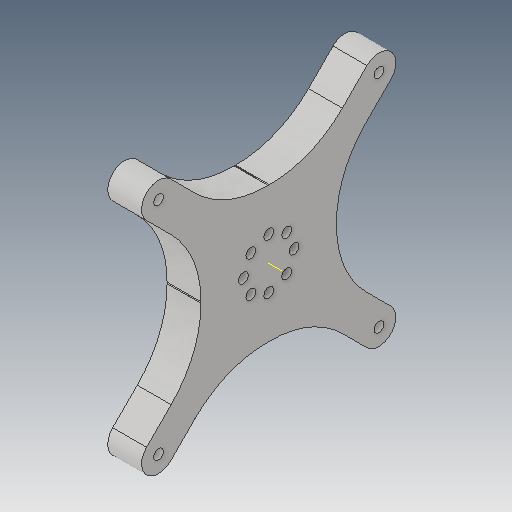
# Autodesk Inventor part: ThrusterMountv2(3)
Saved by Autodesk Inventor 2018 (Build 220112000, 112)
## iProperties
Created: 2019-02-16
Part Number: ThrusterMountv2(3)
Material: Generic
Document SubType Name: Modeling
Designer: anirudh
Density: 1 g/cm^3
Appearance: Default
Mass: 71.9019 g
Surface Area: 161.668 cm^2
Volume: 71.9019 cm^3
Author: anirudh
Autodesk Inventor part; units mm, degrees
ref_plane "YZ Plane" through (0, 0, 0) normal (1, 0, 0) x (0, 1, 0)
ref_plane "XZ Plane" through (0, 0, 0) normal (0, 1, 0) x (-1, 0, 0)
ref_plane "XY Plane" through (0, 0, 0) normal (0, 0, 1) x (1, 0, 0)
sketch "Sketch1" plane through (0, 0, 0) normal (1, 0, 0) x (0, 1, 0)
  circle A0 centre (82.55, 0) radius 1.85
  circle A1 centre (82.55, -82.55) radius 1.85
  circle A2 centre (0, 0) radius 1.85
  circle A3 centre (0, -82.55) radius 1.85
  line L0 (82.55, 0) -> (91.4656, 0) construction
  line L1 (82.55, -82.55) -> (88.8543, -82.55) construction
  arc A4 (54.1751, -19.3947) -> (28.3749, -19.3947) centre (41.275, -41.275) ccw
  arc A5 (19.3947, -28.3749) -> (19.3947, -54.1751) centre (41.275, -41.275) ccw
  arc A6 (28.3749, -63.1553) -> (54.1751, -63.1553) centre (41.275, -41.275) ccw
  arc A7 (63.1553, -54.1751) -> (63.1553, -28.3749) centre (41.275, -41.275) ccw
  arc A8 (87.0401, -4.4901) -> (78.0599, 4.4901) centre (82.55, 0) ccw
  arc A9 (4.4901, 4.4901) -> (-4.4901, -4.4901) centre (0, 0) ccw
  arc A10 (-4.4901, -78.0599) -> (4.4901, -87.0401) centre (0, -82.55) ccw
  arc A11 (78.0599, -87.0401) -> (87.0401, -78.0599) centre (82.55, -82.55) ccw
  line L2 (78.0599, 4.4901) -> (54.1751, -19.3947)
  line L3 (87.0401, -4.4901) -> (63.1553, -28.3749)
  line L4 (87.0401, -78.0599) -> (63.1553, -54.1751)
  line L5 (78.0599, -87.0401) -> (54.1751, -63.1553)
  line L6 (19.3947, -54.1751) -> (-4.4901, -78.0599)
  line L7 (28.3749, -63.1553) -> (4.4901, -87.0401)
  line L8 (19.3947, -28.3749) -> (-4.4901, -4.4901)
  line L9 (4.4901, 4.4901) -> (28.3749, -19.3947)
  circle A12 centre (41.275, -31.775) radius 1.85
  circle A13 centre (50.775, -41.275) radius 1.85
  circle A14 centre (41.275, -50.775) radius 1.85
  circle A15 centre (31.775, -41.275) radius 1.85
  constraints: 20 end point, 16 centre point, 16 point on circle, 6 coincident, 2 horizontal, 1 parallel, 1 perpendicular, 1 tangent
extrude "Extrusion1" add sketch "Sketch1" along normal blind 7.9375
sketch "Sketch2" plane through (0, 0, 0) normal (-1, 0, 0) x (0, 0, 1)
  circle A0 centre (-82.55, 82.55) radius 1.85 projected
  circle A1 centre (-82.55, 82.55) radius 6.35
  arc A2 (4.4901, 78.0599) -> (-4.4901, 87.0401) centre (0, 82.55) ccw projected
  circle A3 centre (0, 82.55) radius 6.35
  circle A4 centre (-82.55, 82.55) radius 1.85
  circle A5 centre (0, 82.55) radius 1.85
  circle A6 centre (0, 0) radius 1.85
  circle A7 centre (0, 0) radius 6.35
  circle A8 centre (-82.55, 0) radius 1.85 projected
  circle A9 centre (-82.55, 0) radius 1.85
  circle A10 centre (-82.55, 0) radius 6.35
  dimension "d24" = 3.7
  constraints: 8 centre point, 8 coincident
  measures "d24" diameter of A4
extrude "Extrusion2" add sketch "Sketch2" along normal blind 7.9375
sketch "Sketch3" plane through (7.9375, 0, 0) normal (1, 0, 0) x (0, 0, -1)
  arc A0 (-4.4901, 4.4901) -> (4.4901, -4.4901) centre (0, 0) ccw
  arc A1 (4.4901, 87.0401) -> (-4.4901, 78.0599) centre (0, 82.55) ccw projected
  arc A2 (4.4901, 87.0401) -> (-4.4901, 78.0599) centre (0, 82.55) ccw
  arc A3 (87.0401, 78.0599) -> (78.0599, 87.0401) centre (82.55, 82.55) ccw projected
  arc A4 (87.0401, 78.0599) -> (78.0599, 87.0401) centre (82.55, 82.55) ccw
  arc A5 (78.0599, -4.4901) -> (87.0401, 4.4901) centre (82.55, 0) ccw projected
  arc A6 (78.0599, -4.4901) -> (87.0401, 4.4901) centre (82.55, 0) ccw
  line L0 (4.4901, 78.0599) -> (0, 73.5697)
  line L1 (-4.4901, 78.0599) -> (19.3947, 54.1751) projected
  line L2 (-4.4901, 78.0599) -> (0, 73.5697)
  line L3 (0, 73.5697) -> (8.9803, 82.55)
  line L4 (28.3749, 63.1553) -> (4.4901, 87.0401) projected
  line L5 (8.9803, 82.55) -> (4.4901, 87.0401)
  line L6 (78.0599, 78.0599) -> (73.5697, 82.55)
  line L7 (73.5697, 82.55) -> (78.0599, 87.0401)
  line L8 (78.0599, 87.0401) -> (73.5697, 82.55)
  line L9 (73.5697, 82.55) -> (82.55, 73.5697)
  line L10 (63.1553, 54.1751) -> (87.0401, 78.0599) projected
  line L11 (82.55, 73.5697) -> (87.0401, 78.0599)
  line L12 (4.4901, 4.4901) -> (0, 8.9803)
  line L13 (19.3947, 28.3749) -> (-4.4901, 4.4901) projected
  line L14 (0, 8.9803) -> (-4.4901, 4.4901)
  line L15 (-4.4901, 4.4901) -> (0, 8.9803)
  line L16 (0, 8.9803) -> (8.9803, 0)
  line L17 (4.4901, -4.4901) -> (28.3749, 19.3947) projected
  line L18 (8.9803, 0) -> (4.4901, -4.4901)
  line L19 (78.0599, 4.4901) -> (73.5697, 0)
  line L20 (73.5697, 0) -> (78.0599, -4.4901)
  line L21 (78.0599, 4.4901) -> (82.55, 8.9803)
  line L22 (87.0401, 4.4901) -> (63.1553, 28.3749) projected
  line L23 (82.55, 8.9803) -> (87.0401, 4.4901)
  constraints: 37 end point, 14 tangent, 13 point on line, 10 point on circle, 9 perpendicular, 4 centre point, 4 coincident, 2 collinear, 2 midpoint, 1 parallel
extrude "Extrusion3" cut sketch "Sketch3" against normal blind 3.175
fillet "Fillet4" radius 38.1 8 edges at (3.9688, 63.1553, -28.3749) (3.9688, 63.1553, -54.1751) (3.9688, 54.1751, -19.3947) (3.9688, 28.3749, -19.3947) (3.9688, 54.1751, -63.1553) (3.9688, 28.3749, -63.1553) (3.9688, 19.3947, -28.3749) (3.9688, 19.3947, -54.1751)
ref_plane "Work Plane1" through (3.9688, 0, 0) normal (1, 0, 0) x (0, 0, -1)
sketch "Sketch6" plane through (3.9688, 0, 0) normal (1, 0, 0) x (0, 0, -1)
  line L0 (18.1155, 56.3523) -> (26.1977, 64.4345) projected
  line L1 (26.1977, 64.4345) -> (18.1155, 56.3523)
  line L2 (36.525, 46.025) -> (18.1155, 56.3523) projected
  line L3 (18.1155, 56.3523) -> (36.525, 46.025)
  line L4 (36.525, 46.025) -> (26.1977, 64.4345)
  line L5 (56.3523, 64.4345) -> (46.025, 46.025) projected
  line L6 (56.3523, 64.4345) -> (46.025, 46.025)
  line L7 (46.025, 46.025) -> (64.4345, 56.3523) projected
  line L8 (46.025, 46.025) -> (64.4345, 56.3523)
  line L9 (56.3523, 64.4345) -> (64.4345, 56.3523) projected
  line L10 (64.4345, 56.3523) -> (56.3523, 64.4345)
  line L11 (18.1155, 26.1977) -> (26.1977, 18.1155) projected
  line L12 (18.1155, 26.1977) -> (26.1977, 18.1155)
  line L13 (36.525, 36.525) -> (26.1977, 18.1155) projected
  line L14 (26.1977, 18.1155) -> (36.525, 36.525)
  line L15 (36.525, 36.525) -> (18.1155, 26.1977)
  line L16 (56.3523, 18.1155) -> (46.025, 36.525) projected
  line L17 (64.4345, 26.1977) -> (56.3523, 18.1155) projected
  line L18 (56.3523, 18.1155) -> (64.4345, 26.1977)
  line L19 (46.025, 36.525) -> (64.4345, 26.1977) projected
  line L20 (64.4345, 26.1977) -> (46.025, 36.525)
  line L21 (46.025, 36.525) -> (56.3523, 18.1155)
  point P0 (0, 0)
  constraints: 24 end point, 9 collinear
extrude "Extrusion5" add sketch "Sketch6" along normal blind 1.27 and the other way blind 3.9688
sketch "Sketch10" plane through (7.9375, 0, 0) normal (1, 0, 0) x (0, 0, -1)
  circle A0 centre (50.775, 41.275) radius 1.85 projected
  circle A1 centre (50.775, 41.275) radius 1.85
  circle A2 centre (41.275, 31.775) radius 1.85 projected
  circle A3 centre (41.275, 31.775) radius 1.85
  circle A4 centre (31.775, 41.275) radius 1.85 projected
  circle A5 centre (31.775, 41.275) radius 1.85
  circle A6 centre (41.275, 50.775) radius 1.85 projected
  circle A7 centre (41.275, 50.775) radius 1.85
  line L0 (82.55, 8.9803) -> (77.8311, 13.6992) projected
  line L1 (68.8508, 4.7189) -> (73.5697, 0) projected
  line L2 (82.55, 8.9803) -> (73.5697, 0)
  line L3 (8.9803, 0) -> (13.6992, 4.7189) projected
  line L4 (4.7189, 13.6992) -> (0, 8.9803) projected
  line L5 (8.9803, 0) -> (0, 8.9803)
  line L6 (82.55, 73.5697) -> (73.5697, 82.55) projected
  line L7 (82.55, 73.5697) -> (73.5697, 82.55)
  line L8 (13.6992, 77.8311) -> (8.9803, 82.55) projected
  line L9 (8.9803, 82.55) -> (0, 73.5697)
  line L10 (77.8311, 68.8508) -> (82.55, 73.5697) projected
  line L11 (82.55, 73.5697) -> (77.8311, 68.8508)
  line L12 (73.5697, 82.55) -> (68.8508, 77.8311) projected
  line L13 (73.5697, 82.55) -> (68.8508, 77.8311)
  line L14 (8.9803, 82.55) -> (0, 73.5697) projected
  line L15 (8.9803, 82.55) -> (13.6992, 77.8311)
  line L16 (0, 73.5697) -> (4.7189, 68.8508) projected
  line L17 (0, 73.5697) -> (4.7189, 68.8508)
  line L18 (0, 8.9803) -> (8.9803, 0) projected
  line L19 (8.9803, 0) -> (13.6992, 4.7189)
  line L20 (0, 8.9803) -> (4.7189, 13.6992)
  line L21 (73.5697, 0) -> (82.55, 8.9803) projected
  line L22 (73.5697, 0) -> (68.8508, 4.7189)
  line L23 (82.55, 8.9803) -> (77.8311, 13.6992)
  arc A8 (41.021, 15.8763) -> (41.529, 15.8763) centre (41.275, 41.275) ccw projected
  line L24 (41.529, 15.8763) -> (41.021, 15.8763)
  arc A9 (15.8763, 41.529) -> (15.8763, 41.021) centre (41.275, 41.275) ccw projected
  line L25 (15.8763, 41.021) -> (15.8763, 41.529)
  arc A10 (41.529, 66.6737) -> (41.021, 66.6737) centre (41.275, 41.275) ccw projected
  line L26 (41.529, 66.6737) -> (41.021, 66.6737)
  arc A11 (66.6737, 41.021) -> (66.6737, 41.529) centre (41.275, 41.275) ccw projected
  line L27 (66.6737, 41.021) -> (66.6737, 41.529)
  arc A12 (68.8508, 4.7189) -> (41.529, 15.8763) centre (41.91, -22.2218) ccw projected
  arc A13 (68.8508, 4.7189) -> (41.529, 15.8763) centre (41.91, -22.2218) ccw
  arc A14 (41.021, 15.8763) -> (13.6992, 4.7189) centre (40.64, -22.2218) ccw
  arc A15 (4.7189, 13.6992) -> (15.8763, 41.021) centre (-23.1549, 41.021) ccw
  arc A16 (15.8763, 41.529) -> (4.7189, 68.8508) centre (-22.2218, 41.91) ccw projected
  arc A17 (15.8763, 41.529) -> (4.7189, 68.8508) centre (-22.2218, 41.91) ccw
  arc A18 (13.6992, 77.8311) -> (41.021, 66.6737) centre (40.64, 104.7718) ccw
  arc A19 (41.529, 66.6737) -> (68.8508, 77.8311) centre (41.91, 104.7718) ccw projected
  arc A20 (41.529, 66.6737) -> (68.8508, 77.8311) centre (41.91, 104.7718) ccw
  arc A21 (77.8311, 68.8508) -> (66.6737, 41.529) centre (104.7718, 41.91) ccw projected
  arc A22 (77.8311, 68.8508) -> (66.6737, 41.529) centre (104.7718, 41.91) ccw
  arc A23 (66.6737, 41.021) -> (77.8311, 13.6992) centre (104.7718, 40.64) ccw
  point P0 (0, 0)
  constraints: 32 end point, 16 point on circle, 12 centre point, 8 collinear, 4 coincident, 3 perpendicular, 3 tangent, 2 horizontal, 2 vertical, 1 point on line
extrude "Extrusion8" cut sketch "Sketch10" against normal blind 3.175
sketch "Sketch11" plane through (7.9375, 41.021, -66.6737) normal (0, 0, 1) x (1, 0, 0)
  line L0 (0, 0.508) -> (-3.175, 0.508) projected
  line L1 (-3.175, 0) -> (0, 0) projected
  line L2 (0, 0.508) -> (-3.175, 0.508)
  line L3 (-3.175, 0.508) -> (-3.175, 0)
  line L4 (-3.175, 0) -> (0, 0)
  line L5 (0, 0) -> (0, 0.508)
  point P0 (-7.9375, -41.021)
  constraints: 8 end point, 2 parallel, 1 horizontal, 1 perpendicular
extrude "Extrusion9" cut sketch "Sketch11" along normal blind 50.8 and the other way blind 25.4
sketch "Sketch12" plane through (7.9375, 15.8763, -41.021) normal (0, 1, 0) x (1, 0, 0)
  line L0 (0, 0) -> (0, 0.508) projected
  line L1 (-3.175, 0.508) -> (0, 0.508) projected
  line L2 (0, 0) -> (-3.175, 0)
  line L3 (-3.175, 0) -> (-3.175, 0.508)
  line L4 (-3.175, 0.508) -> (0, 0.508)
  line L5 (0, 0.508) -> (0, 0)
  point P0 (-7.9375, -41.021)
  constraints: 8 end point, 2 parallel, 1 horizontal, 1 perpendicular
extrude "Extrusion10" cut sketch "Sketch12" along normal blind 53.975 and the other way blind 7.9375
sketch "Sketch13" plane through (4.7625, 0, 0) normal (1, 0, 0) x (0, 0, -1)
  line L0 (41.275, 41.275) -> (41.275, 43.8729)
  circle A0 centre (34.5575, 34.5575) radius 1.85
  circle A1 centre (34.5575, 47.9925) radius 1.85
  circle A2 centre (47.9925, 34.5575) radius 1.85
  circle A3 centre (47.9925, 47.9925) radius 1.85
  point P0 (0, 0)
  point P1 (41.275, 50.775)
  point P2 (41.275, 31.775)
  point P3 (50.775, 41.275)
  constraints: 4 centre point, 2 end point, 1 vertical
extrude "Extrusion12" cut sketch "Sketch13" against normal blind 24.5364
sketch "Sketch15" plane through (0, 0, 0) normal (-1, 0, 0) x (0, 0, 1)
  circle A0 centre (-34.5575, 34.5575) radius 1.85 projected
  circle A1 centre (-34.5575, 34.5575) radius 1.85
  circle A2 centre (-34.5575, 47.9925) radius 1.85 projected
  circle A3 centre (-34.5575, 47.9925) radius 1.85
  circle A4 centre (-47.9925, 47.9925) radius 1.85 projected
  circle A5 centre (-47.9925, 47.9925) radius 1.85
  circle A6 centre (-47.9925, 34.5575) radius 1.85 projected
  circle A7 centre (-47.9925, 34.5575) radius 1.85
  circle A8 centre (-31.775, 41.275) radius 1.85 projected
  circle A9 centre (-31.775, 41.275) radius 1.85
  circle A10 centre (-41.275, 50.775) radius 1.85 projected
  circle A11 centre (-41.275, 50.775) radius 1.85
  circle A12 centre (-50.775, 41.275) radius 1.85 projected
  circle A13 centre (-50.775, 41.275) radius 1.85
  circle A14 centre (-41.275, 31.775) radius 1.85 projected
  circle A15 centre (-41.275, 31.775) radius 1.85
  arc A16 (-4.4901, 87.0401) -> (4.4901, 78.0599) centre (0, 82.55) ccw projected
  circle A17 centre (0, 82.55) radius 6.35
  arc A18 (-78.0599, 87.0401) -> (-87.0401, 78.0599) centre (-82.55, 82.55) ccw projected
  circle A19 centre (-82.55, 82.55) radius 6.35
  arc A20 (-4.4901, -4.4901) -> (4.4901, 4.4901) centre (0, 0) ccw projected
  circle A21 centre (0, 0) radius 6.35
  arc A22 (-87.0401, 4.4901) -> (-78.0599, -4.4901) centre (-82.55, 0) ccw projected
  circle A23 centre (-82.55, 0) radius 6.35
  arc A24 (-66.6737, 41.529) -> (-77.8311, 68.8508) centre (-104.7718, 41.91) ccw projected
  arc A25 (-77.8311, 13.6992) -> (-66.6737, 41.021) centre (-104.7718, 40.64) ccw projected
  line L0 (-87.0401, 4.4901) -> (-77.8311, 13.6992) projected
  arc A26 (-41.021, 66.6737) -> (-41.529, 66.6737) centre (-41.275, 41.275) ccw projected
  line L1 (-41.529, 66.6737) -> (-41.021, 66.6737)
  arc A27 (-15.8763, 41.021) -> (-15.8763, 41.529) centre (-41.275, 41.275) ccw projected
  line L2 (-15.8763, 41.021) -> (-15.8763, 41.529)
  line L3 (-41.021, 15.8763) -> (-41.529, 15.8763)
  line L4 (-66.6737, 41.529) -> (-66.6737, 41.021)
  arc A28 (-66.6771, 41.275) -> (-77.8311, 68.8508) centre (-104.7718, 41.91) ccw
  arc A29 (-77.8311, 13.6992) -> (-66.6771, 41.275) centre (-104.7718, 40.64) ccw
  arc A30 (-13.6992, 4.7189) -> (-41.021, 15.8763) centre (-40.64, -22.2218) ccw projected
  arc A31 (-13.6992, 4.7189) -> (-41.275, 15.8729) centre (-40.64, -22.2218) ccw
  arc A32 (-41.529, 15.8763) -> (-68.8508, 4.7189) centre (-41.91, -22.2218) ccw projected
  arc A33 (-41.275, 15.8729) -> (-68.8508, 4.7189) centre (-41.91, -22.2218) ccw
  arc A34 (-41.021, 66.6737) -> (-13.6992, 77.8311) centre (-40.64, 104.7718) ccw projected
  arc A35 (-41.275, 66.6771) -> (-13.6992, 77.8311) centre (-40.64, 104.7718) ccw
  arc A36 (-68.8508, 77.8311) -> (-41.529, 66.6737) centre (-41.91, 104.7718) ccw projected
  arc A37 (-68.8508, 77.8311) -> (-41.275, 66.6771) centre (-41.91, 104.7718) ccw
  arc A38 (-4.7189, 68.8508) -> (-15.8763, 41.529) centre (22.2218, 41.91) ccw projected
  line L5 (4.4901, 78.0599) -> (-4.7189, 68.8508) projected
  arc A39 (-4.7189, 68.8508) -> (-15.8729, 41.275) centre (22.2218, 41.91) ccw
  arc A40 (-15.8763, 41.021) -> (-4.7189, 13.6992) centre (22.2218, 40.64) ccw projected
  arc A41 (-15.8729, 41.275) -> (-4.7189, 13.6992) centre (22.2218, 40.64) ccw
  line L6 (-4.7189, 13.6992) -> (4.4901, 4.4901) projected
  line L7 (4.4901, 4.4901) -> (-4.7189, 13.6992)
  arc A42 (4.4901, 4.4901) -> (-4.4901, -4.4901) centre (0, 0) ccw projected
  line L8 (-4.4901, -4.4901) -> (-13.6992, 4.7189) projected
  line L9 (-4.4901, -4.4901) -> (-13.6992, 4.7189)
  line L10 (4.4901, 78.0599) -> (-4.7189, 68.8508)
  line L11 (-13.6992, 77.8311) -> (-4.4901, 87.0401) projected
  line L12 (-4.4901, 87.0401) -> (-13.6992, 77.8311)
  arc A43 (-87.0401, 78.0599) -> (-78.0599, 87.0401) centre (-82.55, 82.55) ccw projected
  line L13 (-78.0599, 87.0401) -> (-68.8508, 77.8311) projected
  line L14 (-68.8508, 77.8311) -> (-78.0599, 87.0401)
  line L15 (-77.8311, 68.8508) -> (-87.0401, 78.0599) projected
  line L16 (-77.8311, 68.8508) -> (-87.0401, 78.0599)
  arc A44 (-78.0599, -4.4901) -> (-87.0401, 4.4901) centre (-82.55, 0) ccw projected
  line L17 (-77.8311, 13.6992) -> (-87.0401, 4.4901)
  line L18 (-68.8508, 4.7189) -> (-78.0599, -4.4901) projected
  line L19 (-68.8508, 4.7189) -> (-78.0599, -4.4901)
  constraints: 24 end point, 24 point on circle, 20 coincident, 16 centre point, 15 tangent, 8 collinear, 8 point on line, 2 horizontal, 2 vertical, 15 other
extrude "Extrusion14" add sketch "Sketch15" along normal blind 7.9248 contours A16 L5 A38 A27 A40 L6 A21 L8 A30 L3 A32 L18 A23 L0 A25 L4 A24 L15 A19 L13 A36 A26 A34 L11 | A31 A33 L3
body "Solid1"
